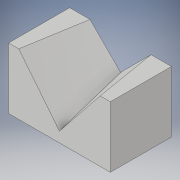
# Autodesk Inventor part: LoftCut
Saved by Autodesk Inventor 2017 (Build 210142000, 142)
## iProperties
Created: 2020-02-11
Part Number: LoftCut
Material: Generic
Document SubType Name: Modeling
Designer: 10042265
Density: 1 g/cm^3
Appearance: Default
Author: 10042265
Autodesk Inventor part; units mm, degrees
ref_plane "YZ Plane" through (0, 0, 0) normal (1, 0, 0) x (0, 1, 0)
ref_plane "XZ Plane" through (0, 0, 0) normal (0, 1, 0) x (-1, 0, 0)
ref_plane "XY Plane" through (0, 0, 0) normal (0, 0, 1) x (1, 0, 0)
sketch "Sketch1" plane through (0, 0, 0) normal (0, 0, 1) x (1, 0, 0)
  line L0 (0, 0) -> (63.5, 0)
  line L1 (63.5, 0) -> (63.5, 38.1)
  line L2 (63.5, 38.1) -> (0, 38.1)
  line L3 (0, 38.1) -> (0, 0)
  dimension "d0" = 63.5
  dimension "d1" = 38.1
  constraints: 8 end point, 3 perpendicular, 1 horizontal
  measures "d0" distance of L0.start L0.end
  measures "d1" distance of L0.end L1.end
extrude "Extrusion1" add sketch "Sketch1" along normal blind 38.1
sketch "Sketch4" plane through (0, 0, 0) normal (0, 0, -1) x (-1, 0, 0)
  line L0 (-31.75, 19.05) -> (-12.7, 38.1)
  line L1 (-31.75, 19.05) -> (-50.8, 38.1)
  line L2 (-50.8, 38.1) -> (-12.7, 38.1)
  point P0 (-63.5, 0)
  constraints: 6 end point, 1 perpendicular
sketch "Sketch3" plane through (0, 0, 38.1) normal (0, 0, 1) x (1, 0, 0)
  line L0 (57.15, 38.1) -> (31.75, 6.35)
  line L1 (31.75, 6.35) -> (6.35, 38.1)
  line L2 (6.35, 38.1) -> (57.15, 38.1)
  point P0 (0, 0)
  point P1 (63.5, 38.1)
  constraints: 6 end point, 1 equal length
loft "Loft1" cut profiles "Sketch4", "Sketch3"
body "Solid1"
